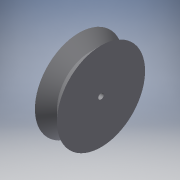
# Autodesk Inventor part: cArmPully
Saved by Autodesk Inventor 2016 SP1 (Build 200210100, 210)
## iProperties
Created: 2016-01-18
Part Number: cArmPully
Material: Generic
Document SubType Name: Modeling
Designer: steele
Density: 1 g/cm^3
Appearance: Default
Author: steele
Autodesk Inventor part; units mm, degrees
ref_plane "YZ Plane" through (0, 0, 0) normal (1, 0, 0) x (0, 1, 0)
ref_plane "XZ Plane" through (0, 0, 0) normal (0, 1, 0) x (-1, 0, 0)
ref_plane "XY Plane" through (0, 0, 0) normal (0, 0, 1) x (1, 0, 0)
sketch "Sketch2" plane through (0, 0, 0) normal (0, 0, 1) x (1, 0, 0)
  line L0 (0, 38.1) -> (-12.7, 50.8)
  line L1 (-12.7, 50.8) -> (-12.7, 0)
  line L2 (-12.7, 0) -> (0, 0)
  line L3 (0, 76.2) -> (0, 0) construction
  line L4 (0, 38.1) -> (12.7, 50.8)
  line L5 (12.7, 50.8) -> (12.7, 0)
  line L6 (12.7, 0) -> (0, 0)
  line L7 (-17.78, 0) -> (17.78, 0) projected
  point P0 (0.5244, 62.9756)
  point P1 (-0.5244, 62.9756)
  dimension "d0" = 45
  dimension "d1" = 50.8
  dimension "d2" = 12.7
  constraints: 14 end point, 3 symmetric about line, 2 vertical, 1 midpoint, 1 perpendicular
  measures "d0" angle of L0 L3
  measures "d1" distance of L1.end L0.end
  measures "d2" distance from line of L2.end L1
revolve "Revolution1" add sketch "Sketch2" angle 360 about axis through (-10, 0, 0) along (1, 0, 0)
sketch "Sketch3" plane through (12.7, 0, 0) normal (1, 0, 0) x (0, 0, -1)
  circle A0 centre (0, 0) radius 3.175
  dimension "d4" = 6.35
  constraints: 1 centre point, 1 coincident
  measures "d4" diameter of A0
extrude "Extrusion1" cut sketch "Sketch3" against normal through all
equation "\"d1\" = pullyRadius"
equation "\"d2\" = 0.5 * pullyWidth"
equation "\"d4\" = boltHoleDiam"
equation "\"pullyDiam\" = 101.6"
equation "\"pullyRadius\" = 0.5 * pullyDiam"
equation "\"pullyWidth\" = 25.4"
equation "\"boltHoleDiam\" = 6.35"
body "Solid1"
